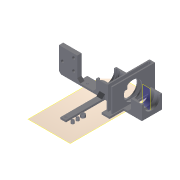
# Autodesk Inventor part: 10_Projector_Base
Saved by Autodesk Inventor 2016 (Build 200138000, 138)
## iProperties
Created: 2017-05-18
Part Number: 10_Projector_Base
Material: Generisch
Document SubType Name: Modeling
Designer: Bene
Density: 1 g/cm^3
Appearance: Vorgabe
Author: Bene
Autodesk Inventor part; units mm, degrees
ref_plane "YZ Plane" through (0, 0, 0) normal (1, 0, 0) x (0, 1, 0)
ref_plane "XZ Plane" through (0, 0, 0) normal (0, 1, 0) x (-1, 0, 0)
ref_plane "XY Plane" through (0, 0, 0) normal (0, 0, 1) x (1, 0, 0)
ref_plane "Arbeitsebene1" through (0, 0, 0) normal (0, 0, 1) x (1, 0, 0)
sketch "Skizze1" plane through (0, 0, 0) normal (0, 0, 1) x (1, 0, 0)
  circle A0 centre (20.3312, 25.1428) radius 3.5 projected
  circle A1 centre (-16.1688, -58.8572) radius 3.5 projected
  circle A2 centre (-27.6688, 22.1428) radius 1.5 projected
  circle A3 centre (1.8312, -42.8572) radius 1.5 projected
  line L0 (-30.1688, -63.8572) -> (11.8312, -63.8572) projected
  line L1 (11.8312, -63.8572) -> (32.8312, -42.8572) projected
  line L2 (32.8312, -42.8572) -> (32.8312, 59.1428) projected
  line L3 (32.8312, 59.1428) -> (-30.1688, 59.1428) projected
  line L4 (-30.1688, 59.1428) -> (-30.1688, -63.8572) projected
  circle A4 centre (-27.6688, 22.1428) radius 2.5
  circle A5 centre (1.8312, -42.8572) radius 2.5
  circle A6 centre (-16.1688, -58.8572) radius 4
  circle A7 centre (20.3312, 25.1428) radius 4
  circle A8 centre (20.3312, 25.1428) radius 1.5
  circle A9 centre (-16.1688, -58.8572) radius 1.5
  point P0 (0, 0)
  dimension "d0" = 1
  dimension "d1" = 1
  dimension "d2" = 0.5
  dimension "d3" = 0.5
  dimension "d37" = 3
  dimension "d38" = 3
  constraints: 6 centre point, 2 coincident
  measures "d0" radial gap between concentric circles of A2 A4
  measures "d1" radial gap between concentric circles of A3 A5
  measures "d2" radial gap between concentric circles of A1 A6
  measures "d3" radial gap between concentric circles of A0 A7
  measures "d37" diameter of A8
  measures "d38" diameter of A9
extrude "Extrusion1" add sketch "Skizze1" along normal blind 4 contours A0 | A4 | A5 | A7
sketch "Skizze2" plane through (-27.6688, 22.1428, 4) normal (0, 0, 1) x (1, 0, 0)
  circle A0 centre (0, 0) radius 1.5 projected
  circle A1 centre (0, 0) radius 2.5 projected
  circle A2 centre (29.5, -65) radius 1.5 projected
  circle A3 centre (29.5, -65) radius 2.5 projected
  circle A4 centre (48, 3) radius 4 projected
  line L0 (-41.5, 1.5) -> (-11.5, 1.5) projected
  line L1 (-11.5, 1.5) -> (-11.5, 43.5) projected
  line L2 (-41.5, 43.5) -> (-11.5, 43.5) projected
  line L3 (-41.5, 1.5) -> (-41.5, 43.5) projected
  line L4 (91.5, 26) -> (89.6246, 26)
  line L5 (91.5, -4) -> (89.6246, -4)
  line L6 (91.5, 26) -> (91.5, -4) projected
  line L7 (22.5, -4) -> (22.5, 26) projected
  line L8 (22.5, 26) -> (24.3754, 26)
  line L9 (22.5, -4) -> (24.3754, -4)
  line L10 (34.2, 11) -> (24.3754, 11) projected
  line L11 (79.8, 11) -> (89.6246, 11) projected
  line L12 (58.5, 44) -> (58.5, 42) construction
  line L13 (58.5, 42) -> (57.5, 42) construction
  line L14 (57.5, 42) -> (57.5, -22) construction
  line L15 (57.5, -22) -> (58.5, -22) construction
  line L16 (58.5, -22) -> (58.5, -26) construction
  line L17 (58.5, -26) -> (59.5, -26) construction
  line L18 (59.5, -26) -> (59.5, -22) construction
  line L19 (59.5, -22) -> (60.5, -22) construction
  line L20 (60.5, -22) -> (60.5, 42) construction
  line L21 (60.5, 42) -> (59.5, 42) construction
  line L22 (59.5, 42) -> (59.5, 44) construction
  line L23 (59.5, 44) -> (58.5, 44) construction
  line L24 (-41.5, 1.5) -> (94.5, 1.5)
  line L25 (94.5, 1.5) -> (94.5, -5.5)
  line L26 (94.5, -5.5) -> (-41.5, -5.5)
  line L27 (-41.5, -5.5) -> (-41.5, 1.5)
  circle A5 centre (29.5, -65) radius 4.5 construction
  line L28 (25, -69.5) -> (34, -69.5)
  line L29 (34, -69.5) -> (34, -5.5)
  line L30 (34, -5.5) -> (25, -5.5)
  line L31 (25, -5.5) -> (25, -69.5)
  line L32 (94.5, 1.5) -> (76.5, 1.5)
  line L33 (76.5, 1.5) -> (76.5, 27.5)
  line L34 (76.5, 27.5) -> (94.5, 27.5)
  line L35 (94.5, 27.5) -> (94.5, 1.5)
  line L36 (19.5, 1.5) -> (37.5, 1.5)
  line L37 (37.5, 1.5) -> (37.5, 27.5)
  line L38 (37.5, 27.5) -> (19.5, 27.5)
  line L39 (19.5, 27.5) -> (19.5, 1.5)
  line L40 (54.5, -25) -> (54.5, 45) construction
  line L41 (54.5, 45) -> (55.5, 45) construction
  line L42 (55.5, 45) -> (55.5, 47) construction
  line L43 (55.5, 47) -> (62.5, 47) construction
  line L44 (62.5, 47) -> (62.5, 45) construction
  line L45 (62.5, 45) -> (63.5, 45) construction
  line L46 (63.5, 45) -> (63.5, -25) construction
  line L47 (63.5, -25) -> (62.5, -25) construction
  line L48 (62.5, -25) -> (62.5, -29) construction
  line L49 (62.5, -29) -> (55.5, -29) construction
  line L50 (55.5, -29) -> (55.5, -25) construction
  line L51 (55.5, -25) -> (54.5, -25) construction
  line L52 (54.5, 47) -> (62.5, 47)
  line L53 (62.5, 47) -> (62.5, -29)
  line L54 (62.5, -29) -> (54.5, -29)
  line L55 (54.5, -29) -> (54.5, 47)
  line L56 (54.5, 47) -> (52, 47)
  line L57 (52, 47) -> (52, -29)
  line L58 (52, -29) -> (54.5, -29)
  line L59 (54.5, -29) -> (54.5, 47)
  line L60 (62.5, 47) -> (65, 47)
  line L61 (65, 47) -> (65, -29)
  line L62 (65, -29) -> (62.5, -29)
  line L63 (62.5, -29) -> (62.5, 47)
  circle A6 centre (48, 3) radius 1.5 projected
  line L64 (76.5, 1.5) -> (65, 1.5)
  line L65 (65, 1.5) -> (65, 11)
  line L66 (65, 11) -> (76.5, 11)
  line L67 (76.5, 11) -> (76.5, 1.5)
  line L68 (37.5, 11) -> (52, 11)
  line L69 (52, 11) -> (52, 1.5)
  line L70 (52, 1.5) -> (37.5, 1.5)
  line L71 (37.5, 1.5) -> (37.5, 11)
  line L72 (19.5, 11) -> (-11.5, 11)
  line L73 (-11.5, 11) -> (-11.5, 1.5)
  line L74 (-11.5, 1.5) -> (19.5, 1.5)
  line L75 (19.5, 1.5) -> (19.5, 11)
  point P0 (27.6688, -22.1428)
  dimension "d6" = 136
  dimension "d7" = 7
  dimension "d8" = 2
  dimension "d9" = 18
  dimension "d10" = 1.5
  dimension "d11" = 18
  dimension "d12" = 3
  dimension "d13" = 3
  dimension "d16" = 2.5
  constraints: 112 end point, 20 parallel, 14 horizontal, 10 perpendicular, 9 point on line, 1 centre point, 17 other
  measures "d6" distance of L25.end L26.end
  measures "d7" distance of L24.end L25.end
  measures "d8" radial gap between concentric circles of A3 A5
  measures "d9" distance of L33.end L34.end
  measures "d10" distance from line of L4.start L34
  measures "d11" distance of L38.end L37.end
  measures "d12" distance between parallel lines of L7 L39
  measures "d13" distance between parallel lines of L14 L40
  measures "d16" distance of L61.end L62.end
extrude "Extrusion2" add sketch "Skizze2" along normal blind 3 contours L24 A1 | L24 A1 | L24 L1 L72 L39 A1 | A1 L24 A4 L57 L26 L27 L0 | L39 L38 L37 L24 | L37 L68 L57 A4 L24 | L26 L29 L28 L31 | L24 A4 | A4 L24 | L57 L24 A4 | L57 L56 L55 L24 | L57 L24 L55 L26 | L26 L55 L58 L57 | L55 L24 L53 L26 | L26 L53 L54 L55 | L55 L52 L53 L24 | L53 L24 L61 L26 | L26 L61 L62 L53 | L53 L60 L61 L24 | L61 L24 L25 L26 | L61 L66 L33 L24 | L33 L34 L35 L24 | A3
sketch "Skizze3" plane through (-27.6688, 22.1428, 7) normal (0, 0, 1) x (1, 0, 0)
  line L0 (58.5, 44) -> (58.5, 42) construction
  line L1 (58.5, 42) -> (57.5, 42) construction
  line L2 (57.5, 42) -> (57.5, -22) construction
  line L3 (57.5, -22) -> (58.5, -22) construction
  line L4 (58.5, -22) -> (58.5, -26) construction
  line L5 (58.5, -26) -> (59.5, -26) construction
  line L6 (59.5, -26) -> (59.5, -22) construction
  line L7 (59.5, -22) -> (60.5, -22) construction
  line L8 (60.5, -22) -> (60.5, 42) construction
  line L9 (60.5, 42) -> (59.5, 42) construction
  line L10 (59.5, 42) -> (59.5, 44) construction
  line L11 (59.5, 44) -> (58.5, 44) construction
  line L12 (56.5, -23) -> (56.5, 43)
  line L13 (56.5, 43) -> (57.5, 43)
  line L14 (57.5, 43) -> (57.5, 45)
  line L15 (57.5, 45) -> (60.5, 45)
  line L16 (60.5, 45) -> (60.5, 43)
  line L17 (60.5, 43) -> (61.5, 43)
  line L18 (61.5, 43) -> (61.5, -23)
  line L19 (61.5, -23) -> (60.5, -23)
  line L20 (60.5, -23) -> (60.5, -27)
  line L21 (60.5, -27) -> (57.5, -27)
  line L22 (57.5, -27) -> (57.5, -23)
  line L23 (57.5, -23) -> (56.5, -23)
  circle A0 centre (0, 0) radius 1.5 projected
  circle A1 centre (29.5, -65) radius 1.5 construction
  line L24 (65, 47) -> (52, 47) projected
  line L25 (52, -5.5) -> (52, -29) projected
  line L26 (-11.5, 1.5) -> (-41.5, 1.5) projected
  line L27 (37.5, 11) -> (37.5, 27.5) projected
  line L28 (37.5, 27.5) -> (19.5, 27.5) projected
  line L29 (19.5, 27.5) -> (19.5, 11) projected
  line L30 (-41.5, 1.5) -> (-41.5, -5.5) projected
  line L31 (-41.5, -5.5) -> (25, -5.5) construction
  line L32 (25, -5.5) -> (25, -69.5) construction
  line L33 (25, -69.5) -> (34, -69.5) construction
  line L34 (34, -69.5) -> (34, -5.5) construction
  line L35 (34, -5.5) -> (52, -5.5) projected
  line L36 (52, -29) -> (65, -29) projected
  line L37 (65, -29) -> (65, -5.5) projected
  line L38 (65, -5.5) -> (94.5, -5.5) construction
  line L39 (94.5, -5.5) -> (94.5, 27.5) projected
  line L40 (94.5, 27.5) -> (76.5, 27.5) projected
  line L41 (76.5, 27.5) -> (76.5, 11) projected
  line L42 (63.5, -25) -> (63.5, 45) construction
  line L43 (63.5, 45) -> (62.5, 45) construction
  line L44 (62.5, 45) -> (62.5, 47) construction
  line L45 (62.5, 47) -> (55.5, 47) construction
  line L46 (55.5, 47) -> (55.5, 45) construction
  line L47 (55.5, 45) -> (54.5, 45) construction
  line L48 (54.5, 45) -> (54.5, -25) construction
  line L49 (54.5, -25) -> (55.5, -25) construction
  line L50 (55.5, -25) -> (55.5, -29) construction
  line L51 (55.5, -29) -> (62.5, -29) construction
  line L52 (62.5, -29) -> (62.5, -25) construction
  line L53 (62.5, -25) -> (63.5, -25) construction
  line L54 (65, 47) -> (52, 47) projected
  line L55 (52, -29) -> (65, -29) projected
  line L56 (54.5, 47) -> (63.5, 47)
  line L57 (63.5, 47) -> (63.5, -29)
  line L58 (63.5, -29) -> (54.5, -29)
  line L59 (54.5, -29) -> (54.5, 47)
  line L60 (54.5, -23) -> (63.5, -23)
  line L61 (63.5, -23) -> (63.5, -29)
  line L62 (63.5, -29) -> (54.5, -29)
  line L63 (54.5, -29) -> (54.5, -23)
  line L64 (19.5, 27.5) -> (37.5, 27.5)
  line L65 (37.5, 27.5) -> (37.5, -5.5)
  line L66 (37.5, -5.5) -> (19.5, -5.5)
  line L67 (19.5, -5.5) -> (19.5, 27.5)
  line L68 (94.5, -5.5) -> (94.5, 27.5) projected
  line L69 (76.5, 27.5) -> (94.5, 27.5)
  line L70 (94.5, 27.5) -> (94.5, -5.5)
  line L71 (94.5, -5.5) -> (76.5, -5.5)
  line L72 (76.5, -5.5) -> (76.5, 27.5)
  line L73 (76.5, 11) -> (65, 11) projected
  line L74 (65, 11) -> (65, 47) projected
  line L75 (52, 47) -> (52, 11) projected
  line L76 (52, 11) -> (37.5, 11) projected
  line L77 (19.5, 11) -> (-11.5, 11) projected
  line L78 (-11.5, 11) -> (-11.5, 1.5) projected
  point P0 (27.6688, -22.1428)
  dimension "d17" = 1
  dimension "d18" = 2
  constraints: 80 end point, 8 parallel, 4 horizontal, 4 perpendicular, 4 point on line, 22 other
  measures "d17" distance between parallel lines of L2 L12
  measures "d18" distance between parallel lines of L18 L42
ref_plane "Arbeitsebene2" through (29.8312, -3.8572, 45.5) normal (0, 0, 1) x (1, 0, 0)
extrude "Extrusion3" add sketch "Skizze3" along normal up to surface (38.5 mm away) contours L60 L59 L24 L57 L18 L17 L16 L15 L14 L13 L12
sketch "Skizze4" plane through (35.8312, -0.8572, 7) normal (1, 0, 0) x (0, 0, -1)
  circle A0 centre (-17, 34) radius 15 projected
  point P0 (7, 0.8572)
extrude "Extrusion4" cut sketch "Skizze4" against normal up to surface (9 mm away)
sketch "Skizze5" plane through (-27.6688, 22.1428, 7) normal (0, 0, 1) x (1, 0, 0)
  line L0 (54.5, -23) -> (54.5, 47) projected
  line L1 (54.5, 47) -> (52, 47) projected
  line L2 (52, -5.5) -> (52, -29) projected
  line L3 (-11.5, 1.5) -> (-41.5, 1.5) projected
  line L4 (37.5, 11) -> (37.5, 27.5) projected
  line L5 (37.5, 27.5) -> (19.5, 27.5) projected
  line L6 (19.5, 27.5) -> (19.5, 11) projected
  line L7 (-41.5, 1.5) -> (-41.5, -5.5) projected
  line L8 (-41.5, -5.5) -> (25, -5.5) projected
  line L9 (25, -5.5) -> (25, -69.5) projected
  line L10 (25, -69.5) -> (34, -69.5) projected
  line L11 (34, -69.5) -> (34, -5.5) projected
  line L12 (34, -5.5) -> (52, -5.5) projected
  line L13 (52, -29) -> (65, -29) projected
  line L14 (65, -29) -> (65, -5.5) projected
  line L15 (65, -5.5) -> (94.5, -5.5) projected
  line L16 (94.5, -5.5) -> (94.5, 27.5) projected
  line L17 (94.5, 27.5) -> (76.5, 27.5) projected
  line L18 (76.5, 27.5) -> (76.5, 11) projected
  line L19 (65, 47) -> (63.5, 47) projected
  line L20 (63.5, 47) -> (63.5, -23) projected
  line L21 (63.5, -23) -> (61.5, -23) projected
  line L22 (61.5, -23) -> (61.5, 43) projected
  line L23 (61.5, 43) -> (60.5, 43) projected
  line L24 (60.5, 43) -> (60.5, 45) projected
  line L25 (60.5, 45) -> (57.5, 45) projected
  line L26 (57.5, 45) -> (57.5, 43) projected
  line L27 (57.5, 43) -> (56.5, 43) projected
  line L28 (56.5, 43) -> (56.5, -23) projected
  line L29 (56.5, -23) -> (54.5, -23) projected
  circle A0 centre (0, 0) radius 1.5 projected
  circle A1 centre (29.5, -65) radius 1.5 projected
  line L30 (19.5, 27.5) -> (37.5, 27.5)
  line L31 (37.5, 27.5) -> (37.5, -5.5)
  line L32 (37.5, -5.5) -> (19.5, -5.5)
  line L33 (19.5, -5.5) -> (19.5, 27.5)
  line L34 (76.5, 27.5) -> (94.5, 27.5)
  line L35 (94.5, 27.5) -> (94.5, -5.5)
  line L36 (94.5, -5.5) -> (76.5, -5.5)
  line L37 (76.5, -5.5) -> (76.5, 27.5)
  line L38 (52, 47) -> (52, 11) projected
  line L39 (52, 11) -> (37.5, 11) projected
  line L40 (19.5, 11) -> (-11.5, 11) projected
  line L41 (-11.5, 11) -> (-11.5, 1.5) projected
  line L42 (76.5, 11) -> (65, 11) projected
  line L43 (65, 11) -> (65, 47) projected
  point P0 (27.6688, -22.1428)
  constraints: 16 end point, 4 parallel, 2 horizontal, 2 perpendicular, 1 point on line
extrude "Extrusion5" add sketch "Skizze5" along normal blind 20 contours L31 L12 L32 L8 L33 L6 L5 L4 | L37 L18 L17 L16 L15
ref_plane "Arbeitsebene3" through (58.0812, 33.1428, 24) normal (0, 1, 0) x (1, 0, 0)
sketch "Skizze6" plane through (58.0812, 33.1428, 24) normal (0, 1, 0) x (1, 0, 0)
  spline S0 degree 4 poles (-51.55, 0) (-51.55, -0.0682) (-51.5513, -0.2064) (-51.557, -0.5152) (-51.5723, -0.787) (-51.5953, -1.1366) (-51.6258, -1.442) (-51.6734, -1.851) (-51.7335, -2.2429) (-51.8059, -2.6431) (-51.8905, -3.0347) (-51.9653, -3.3492) (-52.0677, -3.7381) (-52.2045, -4.2021) (-52.384, -4.7365) (-52.6153, -5.3382) (-52.8718, -5.9294) (-53.1524, -6.5098) (-53.4557, -7.0784) (-53.7808, -7.6349) (-54.1314, -8.1869) (-54.5934, -8.8584) (-55.1837, -9.6359) (-55.8166, -10.3802) (-56.4786, -11.0841) (-57.0531, -11.6499) (-57.5232, -12.0887) (-58.1287, -12.6239) (-58.7455, -13.1345) (-59.3893, -13.6321) (-60.0304, -14.0996) (-60.5112, -14.4328) (-60.88, -14.6809) (-61.1998, -14.8882) (-61.317, -14.9634) (-61.3746, -15) knots 0.068021 0.068021 0.068021 0.068021 0.068021 0.082601 0.097181 0.111761 0.126341 0.140921 0.155501 0.184661 0.199241 0.213821 0.228401 0.242981 0.272141 0.301301 0.330461 0.359621 0.388781 0.41794 0.4471 0.47626 0.507128 0.565447 0.623767 0.652927 0.682087 0.711247 0.740407 0.798727 0.827887 0.857047 0.886207 0.900787 0.915367 0.915367 0.915367 0.915367 0.915367 construction
  spline S1 degree 4 poles (-5.95, 0) (-5.95, -0.0682) (-5.9487, -0.2064) (-5.943, -0.5152) (-5.9277, -0.787) (-5.9047, -1.1366) (-5.8742, -1.442) (-5.8266, -1.851) (-5.7665, -2.2429) (-5.6941, -2.6431) (-5.6095, -3.0347) (-5.5347, -3.3492) (-5.4323, -3.7381) (-5.2955, -4.2021) (-5.116, -4.7365) (-4.8847, -5.3382) (-4.6282, -5.9294) (-4.3476, -6.5098) (-4.0443, -7.0784) (-3.7192, -7.6349) (-3.3686, -8.1869) (-2.9066, -8.8584) (-2.3163, -9.6359) (-1.6834, -10.3802) (-1.0214, -11.0841) (-0.4469, -11.6499) (0.0232, -12.0887) (0.6287, -12.6239) (1.2455, -13.1345) (1.8893, -13.6321) (2.5304, -14.0996) (3.0112, -14.4328) (3.38, -14.6809) (3.6998, -14.8882) (3.817, -14.9634) (3.8746, -15) knots 0.068021 0.068021 0.068021 0.068021 0.068021 0.082601 0.097181 0.111761 0.126341 0.140921 0.155501 0.184661 0.199241 0.213821 0.228401 0.242981 0.272141 0.301301 0.330461 0.359621 0.388781 0.41794 0.4471 0.47626 0.507128 0.565447 0.623767 0.652927 0.682087 0.711247 0.740407 0.798727 0.827887 0.857047 0.886207 0.900787 0.915367 0.915367 0.915367 0.915367 0.915367 projected
  line L0 (5.75, 15) -> (5.75, -15) projected
  spline S2 degree 4 poles (-5.95, 0) (-5.95, 0.0682) (-5.9487, 0.2064) (-5.943, 0.5152) (-5.9277, 0.787) (-5.9047, 1.1366) (-5.8742, 1.442) (-5.8266, 1.851) (-5.7665, 2.2429) (-5.6941, 2.6431) (-5.6095, 3.0347) (-5.5347, 3.3492) (-5.4323, 3.7381) (-5.2955, 4.2021) (-5.116, 4.7365) (-4.8847, 5.3382) (-4.6282, 5.9294) (-4.3476, 6.5098) (-4.0443, 7.0784) (-3.7192, 7.6349) (-3.3686, 8.1869) (-2.9066, 8.8584) (-2.3163, 9.6359) (-1.6834, 10.3802) (-1.0214, 11.0841) (-0.4469, 11.6499) (0.0232, 12.0887) (0.6287, 12.6239) (1.2455, 13.1345) (1.8893, 13.6321) (2.5304, 14.0996) (3.0112, 14.4328) (3.38, 14.6809) (3.6998, 14.8882) (3.817, 14.9634) (3.8746, 15) knots 0.068021 0.068021 0.068021 0.068021 0.068021 0.082601 0.097181 0.111761 0.126341 0.140921 0.155501 0.184661 0.199241 0.213821 0.228401 0.242981 0.272141 0.301301 0.330461 0.359621 0.388781 0.41794 0.4471 0.47626 0.507128 0.565447 0.623767 0.652927 0.682087 0.711247 0.740407 0.798727 0.827887 0.857047 0.886207 0.900787 0.915367 0.915367 0.915367 0.915367 0.915367 projected
  spline S3 degree 4 poles (-5.95, 0) (-5.95, -0.0682) (-5.9487, -0.2064) (-5.943, -0.5152) (-5.9277, -0.787) (-5.9047, -1.1366) (-5.8742, -1.442) (-5.8266, -1.851) (-5.7665, -2.2429) (-5.6941, -2.6431) (-5.6095, -3.0347) (-5.5347, -3.3492) (-5.4323, -3.7381) (-5.2955, -4.2021) (-5.116, -4.7365) (-4.8847, -5.3382) (-4.6282, -5.9294) (-4.3476, -6.5098) (-4.0443, -7.0784) (-3.7192, -7.6349) (-3.3686, -8.1869) (-2.9066, -8.8584) (-2.3163, -9.6359) (-1.6834, -10.3802) (-1.0214, -11.0841) (-0.4469, -11.6499) (0.0232, -12.0887) (0.6287, -12.6239) (1.2455, -13.1345) (1.8893, -13.6321) (2.5304, -14.0996) (3.0112, -14.4328) (3.38, -14.6809) (3.6998, -14.8882) (3.817, -14.9634) (3.8746, -15) knots 0.068021 0.068021 0.068021 0.068021 0.068021 0.082601 0.097181 0.111761 0.126341 0.140921 0.155501 0.184661 0.199241 0.213821 0.228401 0.242981 0.272141 0.301301 0.330461 0.359621 0.388781 0.41794 0.4471 0.47626 0.507128 0.565447 0.623767 0.652927 0.682087 0.711247 0.740407 0.798727 0.827887 0.857047 0.886207 0.900787 0.915367 0.915367 0.915367 0.915367 0.915367 projected
  spline S4 degree 4 poles (-5.95, 0) (-5.95, -0.0682) (-5.9487, -0.2064) (-5.943, -0.5152) (-5.9277, -0.787) (-5.9047, -1.1366) (-5.8742, -1.442) (-5.8266, -1.851) (-5.7665, -2.2429) (-5.6941, -2.6431) (-5.6095, -3.0347) (-5.5347, -3.3492) (-5.4323, -3.7381) (-5.2955, -4.2021) (-5.116, -4.7365) (-4.8847, -5.3382) (-4.6282, -5.9294) (-4.3476, -6.5098) (-4.0443, -7.0784) (-3.7192, -7.6349) (-3.3686, -8.1869) (-2.9066, -8.8584) (-2.3163, -9.6359) (-1.6834, -10.3802) (-1.0214, -11.0841) (-0.4469, -11.6499) (0.0232, -12.0887) (0.6287, -12.6239) (1.2455, -13.1345) (1.8893, -13.6321) (2.5304, -14.0996) (3.0112, -14.4328) (3.38, -14.6809) (3.6998, -14.8882) (3.817, -14.9634) (3.8746, -15) knots 0.068021 0.068021 0.068021 0.068021 0.068021 0.082601 0.097181 0.111761 0.126341 0.140921 0.155501 0.184661 0.199241 0.213821 0.228401 0.242981 0.272141 0.301301 0.330461 0.359621 0.388781 0.41794 0.4471 0.47626 0.507128 0.565447 0.623767 0.652927 0.682087 0.711247 0.740407 0.798727 0.827887 0.857047 0.886207 0.900787 0.915367 0.915367 0.915367 0.915367 0.915367 projected
  spline S5 degree 4 poles (-5.95, 0) (-5.95, 0.0682) (-5.9487, 0.2064) (-5.943, 0.5152) (-5.9277, 0.787) (-5.9047, 1.1366) (-5.8742, 1.442) (-5.8266, 1.851) (-5.7665, 2.2429) (-5.6941, 2.6431) (-5.6095, 3.0347) (-5.5347, 3.3492) (-5.4323, 3.7381) (-5.2955, 4.2021) (-5.116, 4.7365) (-4.8847, 5.3382) (-4.6282, 5.9294) (-4.3476, 6.5098) (-4.0443, 7.0784) (-3.7192, 7.6349) (-3.3686, 8.1869) (-2.9066, 8.8584) (-2.3163, 9.6359) (-1.6834, 10.3802) (-1.0214, 11.0841) (-0.4469, 11.6499) (0.0232, 12.0887) (0.6287, 12.6239) (1.2455, 13.1345) (1.8893, 13.6321) (2.5304, 14.0996) (3.0112, 14.4328) (3.38, 14.6809) (3.6998, 14.8882) (3.817, 14.9634) (3.8746, 15) knots 0.068021 0.068021 0.068021 0.068021 0.068021 0.082601 0.097181 0.111761 0.126341 0.140921 0.155501 0.184661 0.199241 0.213821 0.228401 0.242981 0.272141 0.301301 0.330461 0.359621 0.388781 0.41794 0.4471 0.47626 0.507128 0.565447 0.623767 0.652927 0.682087 0.711247 0.740407 0.798727 0.827887 0.857047 0.886207 0.900787 0.915367 0.915367 0.915367 0.915367 0.915367 projected
  line L1 (5.75, 15) -> (5.75, -15) projected
  line L2 (5.75, -15) -> (3.8746, -15)
  line L3 (-63.25, 0) -> (-51.55, 0) construction
  line L4 (-73.1079, 0) -> (21.6589, 0)
  line L5 (-63.25, 0) -> (-72.6894, 0) construction
  line L6 (-72.6894, 0) -> (-72.6894, 13.0329) construction
  line L7 (-72.6894, 13.0329) -> (-63.5278, 13.0329) construction
  line L8 (-58.63, 13.0329) -> (-46.8646, 13.0329) construction
  line L9 (-46.8646, 13.0329) -> (-46.8646, 0) construction
  line L10 (-46.8646, 0) -> (-58.63, 0) construction
  line L11 (-58.63, 0) -> (-58.63, 13.0329) construction
  line L12 (-72.6894, 0) -> (-46.8646, 0)
  line L13 (-46.8646, 0) -> (-46.8646, 13.0329)
  line L14 (-46.8646, 13.0329) -> (-57.5807, 13.0329)
  line L15 (-72.6894, 0) -> (-72.6894, 13.0329)
  line L16 (-72.6894, 13.0329) -> (-63.5278, 13.0329)
  arc A0 (-57.5807, 13.0329) -> (-60.6208, 15.3932) centre (-73.8332, -4.763) ccw
  line L17 (-12.9854, 0) -> (-12.9854, 13.0329)
  line L18 (-12.9854, 13.0329) -> (-0.4058, 13.0329)
  line L19 (16.9111, 0) -> (16.9111, 13.0329)
  line L20 (16.9111, 13.0329) -> (5.75, 13.0329)
  line L21 (5.75, 13.0329) -> (5.75, 15.3427)
  line L22 (5.75, 15.3427) -> (3.2205, 15.3427)
  arc A1 (3.2205, 15.3427) -> (-0.4058, 13.0329) centre (5.8773, 7.1699) ccw
  line L23 (-63.5278, 13.0329) -> (-63.5278, 15.3932)
  line L24 (-63.5278, 15.3932) -> (-60.6208, 15.3932)
  point P0 (-58.0812, 24)
  point P1 (-63.25, -15)
  constraints: 46 end point, 7 perpendicular, 7 point on line, 5 horizontal, 4 point on circle, 3 collinear, 3 parallel, 3 vertical, 2 centre point, 2 coincident, 3 other
revolve "Umdrehung2" cut sketch "Skizze6" angle 360 about axis through (-15.0267, 33.1428, 24) along (1, 0, 0) contours L4 L17 L18 A1 L22 L21 L0 | L0 L20 L19 L4 | L15 L16 L23 L24 A0 L14 L13 L4
sketch "Skizze7" plane through (-27.6688, 22.1428, 7) normal (0, 0, 1) x (1, 0, 0)
  line L0 (-41.5, 1.5) -> (-11.5, 1.5) projected
  line L1 (-11.5, 1.5) -> (-11.5, 43.5) projected
  line L2 (-41.5, 43.5) -> (-11.5, 43.5) projected
  line L3 (-41.5, 1.5) -> (-41.5, 43.5) projected
  line L4 (-41.5, 1.5) -> (-41.5, -5.5) projected
  line L5 (-41.5, -5.5) -> (-11.5, -5.5)
  line L6 (-11.5, -5.5) -> (-11.5, 1.5)
  line L7 (-11.5, 1.5) -> (-41.5, 1.5)
  line L8 (-41.5, 1.5) -> (-41.5, -5.5)
  point P0 (27.6688, -22.1428)
  constraints: 8 end point, 2 parallel, 1 horizontal, 1 perpendicular
ref_plane "Arbeitsebene4" through (-69.1688, 23.6428, 44) normal (0, 0, 1) x (1, 0, 0)
extrude "Extrusion6" add sketch "Skizze7" along normal up to surface (37 mm away) contours L0 L6 L5 L4
sketch "Skizze8" plane through (-69.1688, 16.6428, 4) normal (0, -1, 0) x (1, 0, 0)
  circle A0 centre (24, 15.5) radius 1.5 projected
  circle A1 centre (24, 34) radius 1.5 projected
  circle A2 centre (5.5, 20) radius 1.5 projected
  line L0 (0, 0) -> (0, 40) projected
  line L1 (0, 40) -> (30, 40) projected
  line L2 (30, 40) -> (30, 0) projected
  line L3 (30, 0) -> (0, 0) projected
  circle A3 centre (24, 34) radius 2.5
  circle A4 centre (24, 15.5) radius 2.5
  circle A5 centre (5.5, 20) radius 2.5
  point P0 (69.1688, -4)
  dimension "d29" = 1
  dimension "d30" = 1
  dimension "d31" = 1
  constraints: 3 centre point
  measures "d29" radial gap between concentric circles of A1 A3
  measures "d30" radial gap between concentric circles of A0 A4
  measures "d31" radial gap between concentric circles of A2 A5
extrude "Extrusion7" cut sketch "Skizze8" against normal through all contours A0 | A1 | A2 | A3 | A4 | A5
chamfer "Fase1" distance 5 angle 45 5 edges at (-8.1688, 24.8928, 7) (1.8312, 16.6428, 7) (-39.1688, 20.1428, 7) (9.8312, 24.8928, 7) (48.8312, 24.8928, 7)
sketch "Skizze9" plane through (1.8312, -42.8572, 0) normal (0, 0, -1) x (-1, 0, 0)
  circle A0 centre (0, 0) radius 2.5 projected
  circle A1 centre (0, 0) radius 1.5 projected
  circle A2 centre (-18.5, 68) radius 1.5 projected
  circle A3 centre (-18.5, 68) radius 4 projected
  circle A4 centre (29.5, 65) radius 1.5 projected
  circle A5 centre (29.5, 65) radius 2.5 projected
  point P0 (1.8312, 42.8572)
extrude "Extrusion8" cut sketch "Skizze9" against normal up to surface (4 mm away)
sketch "Skizze10" plane through (-27.6688, 22.1428, 4) normal (0, 0, -1) x (-1, 0, 0)
  circle A0 centre (-29.5, -65) radius 1.5 projected
  circle A1 centre (-48, 3) radius 3.5 projected
  circle A2 centre (-48, 3) radius 1.5 projected
  circle A3 centre (-40.495, -65) radius 1.5
  circle A4 centre (-40.495, -56.8575) radius 1.5
  circle A5 centre (-40.495, -65) radius 2.5
  circle A6 centre (-40.495, -56.8575) radius 2.5
  circle A7 centre (-40.0763, -47.6744) radius 3.5
  circle A8 centre (-40.0763, -47.6744) radius 2
  point P0 (-27.6688, -22.1428)
  dimension "d41" = 3
  dimension "d42" = 3
  dimension "d43" = 1
  dimension "d44" = 1
  dimension "d47" = 7
  dimension "d51" = 4
  constraints: 6 centre point, 1 coincident
  measures "d41" diameter of A3
  measures "d42" diameter of A4
  measures "d43" radial gap between concentric circles of A3 A5
  measures "d44" radial gap between concentric circles of A4 A6
  measures "d47" diameter of A7
  measures "d51" diameter of A8
extrude "Extrusion9" add sketch "Skizze10" against normal blind 4 contours A5 | A6 | A7
